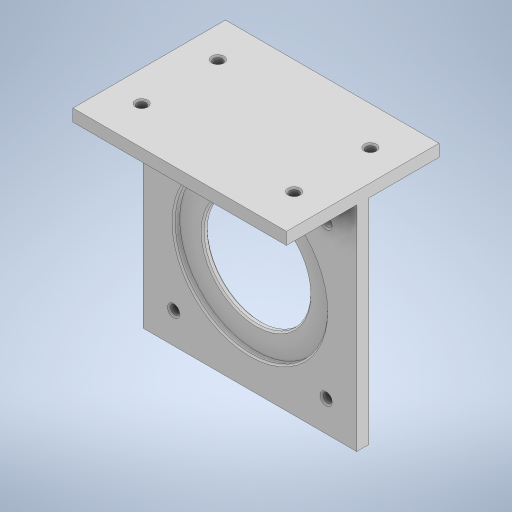
# Autodesk Inventor part: Кронштейн мотора
Saved by Autodesk Inventor 2023 (Build 270158000, 158)
## iProperties
Created: 2022-05-17
Part Number: Кронштейн мотора
Material: Типовые
Document SubType Name: Modeling
Designer: avkap
Density: 1 g/cm^3
Appearance: По умолчанию
Author: avkap
Autodesk Inventor part; units mm, degrees
ref_plane "YZ Plane" through (0, 0, 0) normal (1, 0, 0) x (0, 1, 0)
ref_plane "XZ Plane" through (0, 0, 0) normal (0, 1, 0) x (-1, 0, 0)
ref_plane "XY Plane" through (0, 0, 0) normal (0, 0, 1) x (1, 0, 0)
sketch "Эскиз1" plane through (0, 0, 0) normal (0, 0, 1) x (1, 0, 0)
  line L0 (0, 0) -> (140, 0)
  line L1 (140, 0) -> (140, 140)
  line L2 (140, 140) -> (0, 140)
  line L3 (0, 140) -> (0, 0)
  circle A0 centre (70, 70) radius 50
  line L4 (0, 140) -> (20, 140)
  line L5 (20, 140) -> (20, 120)
  line L6 (140, 0) -> (140, 20)
  line L7 (140, 20) -> (120, 20)
  line L8 (20, 120) -> (120, 120)
  line L9 (120, 120) -> (120, 20)
  line L10 (120, 20) -> (20, 20)
  line L11 (20, 20) -> (20, 120)
  line L12 (70, 70) -> (0, 70)
  line L13 (0, 70) -> (0, 0)
  line L14 (0, 0) -> (70, 0)
  line L15 (70, 0) -> (70, 70)
  circle A1 centre (20, 120) radius 3
  circle A2 centre (120, 120) radius 3
  circle A3 centre (120, 20) radius 3
  circle A4 centre (20, 20) radius 3
  dimension "d0" = 140
  dimension "d1" = 140
  dimension "d2" = 100
  dimension "d3" = 20
  dimension "d4" = 20
  dimension "d5" = 20
  dimension "d6" = 20
  dimension "d7" = 70
  dimension "d8" = 70
  dimension "d9" = 6
  dimension "d10" = 6
  dimension "d11" = 6
  dimension "d14" = 6
  constraints: 32 end point, 6 parallel, 5 centre point, 5 perpendicular, 4 coincident, 3 horizontal, 2 point on line
  measures "d0" distance of L2.end L1.end
  measures "d1" distance of L1.end L0.end
  measures "d2" diameter of A0
  measures "d3" distance of L2.end L4.end
  measures "d4" distance of L4.end L5.end
  measures "d5" distance of L0.end L6.end
  measures "d6" distance of L6.end L7.end
  measures "d7" distance of L0.start L14.end
  measures "d8" distance of L14.end L12.start
  measures "d9" diameter of A1
  measures "d10" diameter of A2
  measures "d11" diameter of A3
  measures "d14" diameter of A4
extrude "Выдавливание1" add sketch "Эскиз1" along normal blind 4 contours L3 L12 L11 A4 L10 L15 L0 | L15 L10 A3 L7 L1 L0 | L3 L2 L5 A1 L11 L12 | L10 A4 L11 A0 | A0 L9 A3 L10 | L11 A1 L8 A0 | L7 A3 L9 A2 L8 A1 L5 L2 L1 | A0 L8 A2 L9
sketch "Эскиз2" plane through (0, 140, 0) normal (0, 1, 0) x (1, 0, 0)
  line L0 (0, 0) -> (0, -4) projected
  line L1 (0, 0) -> (140, 0)
  line L2 (140, 0) -> (140, -50)
  line L3 (140, -50) -> (0, -50)
  line L4 (0, -50) -> (0, 0)
  line L5 (0, -25) -> (20, -25)
  line L6 (140, -25) -> (120, -25)
  circle A0 centre (120, -25) radius 3
  circle A1 centre (20, -25) radius 3
  line L7 (140, 0) -> (0, 0)
  line L8 (0, 0) -> (0, 50)
  line L9 (0, 50) -> (140, 50)
  line L10 (140, 50) -> (140, 0)
  line L11 (140, 25) -> (120, 25)
  circle A2 centre (120, 25) radius 3
  circle A3 centre (20, 25) radius 3
  line L12 (0, 25) -> (20, 25)
  point P0 (0, -4)
  point P1 (0, 0)
  dimension "d15" = 140
  dimension "d16" = 50
  dimension "d17" = 20
  dimension "d18" = 20
  dimension "d19" = 6
  dimension "d20" = 6
  dimension "d23" = 140
  dimension "d24" = 50
  dimension "d25" = 6
  dimension "d26" = 6
  dimension "d30" = 20
  constraints: 24 end point, 5 horizontal, 4 centre point, 4 coincident, 4 midpoint, 4 parallel, 2 perpendicular, 1 point on line
  measures "d15" distance of L2.end L3.end
  measures "d16" distance of L1.end L2.end
  measures "d17" distance of L5.start L5.end
  measures "d18" distance of L6.start L6.end
  measures "d19" diameter of A0
  measures "d20" diameter of A1
  measures "d23" distance of L8.end L9.end
  measures "d24" distance of L7.end L8.end
  measures "d25" diameter of A2
  measures "d26" diameter of A3
  measures "d30" distance of L12.start L12.end
extrude "Выдавливание2" add sketch "Эскиз2" along normal blind 8
sketch "Эскиз3" plane through (0, 0, 0) normal (0, 0, -1) x (-1, 0, 0)
  line L0 (0, 0) -> (-140, 0) projected
  line L1 (-140, 140) -> (0, 140) projected
  line L2 (-140, 0) -> (0, 0)
  line L3 (0, 0) -> (0, 140)
  line L4 (0, 140) -> (-140, 140)
  line L5 (-140, 140) -> (-140, 0)
  circle A0 centre (-120, 20) radius 3 projected
  circle A1 centre (-120, 120) radius 3 projected
  circle A2 centre (-20, 120) radius 3 projected
  circle A3 centre (-20, 20) radius 3 projected
  circle A4 centre (-70, 70) radius 35
  circle A5 centre (-70, 70) radius 50 projected
  dimension "d27" = 70
  constraints: 8 end point, 2 parallel, 1 centre point, 1 horizontal, 1 perpendicular
  measures "d27" diameter of A4
extrude "Выдавливание3" add sketch "Эскиз3" along normal blind 4 contours L0 L5 L1 L3 | A5
chamfer "Фаска1" distance 1 angle 45 19 edges at (23, 20, -4) (105, 70, -4) (123, 20, -4) (123, 120, -4) (117, 140, -25) (17, 140, -25) (23, 120, -4) (20, 70, 4) (105, 70, 0) (117, 120, 4) (117, 140, 25) (17, 140, 25) (17, 120, 4) (17, 20, 4) (117, 20, 4) (17, 148, 25) (17, 148, -25) (117, 148, 25) (117, 148, -25)
